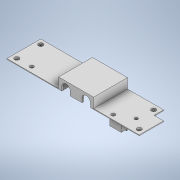
# Autodesk Inventor part: Klapa_kanalpow
Saved by Autodesk Inventor 2022 (Build 260153000, 153)
## iProperties
Created: 2022-09-09
Part Number: Klapa_kanalpow
Material: Ogólny
Document SubType Name: Modeling
Designer: kosak
Density: 1 g/cm^3
Appearance: Domyślna
Author: kosak
Autodesk Inventor part; units mm, degrees
ref_plane "YZ Plane" through (0, 0, 0) normal (1, 0, 0) x (0, 1, 0)
ref_plane "XZ Plane" through (0, 0, 0) normal (0, 1, 0) x (-1, 0, 0)
ref_plane "XY Plane" through (0, 0, 0) normal (0, 0, 1) x (1, 0, 0)
sketch "Szkic1" plane through (0, 0, 0) normal (0, 1, 0) x (-1, 0, 0)
  line L0 (0, 0) -> (174, 0)
  line L1 (174, 0) -> (174, -44.5)
  line L2 (174, -44.5) -> (12.5, -44.5)
  line L3 (0, -32) -> (0, 0)
  line L4 (0, -44.5) -> (12.5, -44.5)
  line L5 (12.5, -44.5) -> (12.5, -32)
  line L6 (12.5, -32) -> (0, -32)
  line L7 (0, -32) -> (0, -44.5)
  dimension "d0" = 174
  dimension "d1" = 44.5
  dimension "d9" = 12.5
  dimension "d10" = 12.5
  constraints: 16 end point, 4 parallel, 2 horizontal, 2 perpendicular
  measures "d0" distance of L1.end L4.start
  measures "d1" distance of L0.end L1.end
  measures "d9" distance of L3.start L5.end
  measures "d10" distance of L2.end L5.end
extrude "Wyciągnięcie proste1" add sketch "Szkic1" along normal blind 1 contours L0 L1 L2 L5 L6 L3
sketch "Szkic2" plane through (0, 0, 0) normal (0, -1, 0) x (1, 0, 0)
  line L0 (-12.5, -44.5) -> (-174, -44.5) projected
  line L1 (0, 0) -> (0, -32) projected
  line L2 (-174, 0) -> (0, 0) projected
  line L3 (-174, -44.5) -> (-174, 0) projected
  line L4 (-171, -41.5) -> (-15, -41.5)
  line L5 (-3, -29.5) -> (-3, -3)
  line L6 (-3, -3) -> (-171, -3)
  line L7 (-171, -3) -> (-171, -41.5)
  line L8 (-12.5, -44.5) -> (-174, -44.5) projected
  line L9 (-15, -41.5) -> (-15, -29.5)
  line L10 (-15, -29.5) -> (-3, -29.5)
  line L11 (-12.5, -32) -> (-12.5, -44.5) projected
  line L12 (0, -32) -> (-12.5, -32) projected
  dimension "d4" = 3
  dimension "d6" = 12
  dimension "d11" = 12
  constraints: 12 end point, 1 other
  measures "d4" distance between parallel lines of L0 L4
  measures "d6" distance of L4.end L9.end
  measures "d11" distance of L9.end L5.start
extrude "Wyciągnięcie proste2" add sketch "Szkic2" along normal blind 2 contours L7 L6 L5 L10 L9 L4
sketch "Szkic4" plane through (0, 1, 0) normal (0, 1, 0) x (1, 0, 0)
  line L0 (-174, 44.5) -> (-174, 0) projected
  line L1 (-174, 22.25) -> (-106, 22.25)
  line L2 (0, 22.25) -> (-60, 22.25)
  line L3 (0, 0) -> (0, 32) projected
  line L4 (-60, 0) -> (-106, 0)
  line L5 (-106, 0) -> (-106, 44.5)
  line L6 (-106, 44.5) -> (-60, 44.5)
  line L7 (-60, 44.5) -> (-60, 0)
  line L8 (-174, 0) -> (0, 0) projected
  line L9 (-12.5, 44.5) -> (-174, 44.5) projected
  dimension "d24" = 60
  dimension "d51" = 68
  constraints: 12 end point, 3 midpoint, 2 collinear, 2 horizontal, 1 parallel, 1 perpendicular, 1 point on line
  measures "d24" distance of L2.start L2.end
  measures "d51" distance of L1.end L1.start
extrude "Wyciągnięcie proste4" add sketch "Szkic4" along normal blind 13 contours L6 L7 L4 L5
sketch "Szkic9" plane through (0, -2, 0) normal (0, -1, 0) x (1, 0, 0)
  line L0 (-60, -44.5) -> (-60, 0) projected
  line L1 (-106, 0) -> (-106, -44.5) projected
  line L2 (-12.5, -44.5) -> (-174, -44.5) projected
  line L3 (-174, 0) -> (0, 0) projected
  line L4 (-104, 0) -> (-104, -44.5)
  line L5 (-62, -44.5) -> (-62, 0)
  line L6 (-12.5, -42.5) -> (-174, -42.5)
  line L7 (-174, -2) -> (0, -2)
  line L8 (-62, -2) -> (-104, -2)
  line L9 (-104, -2) -> (-104, -42.5)
  line L10 (-104, -42.5) -> (-62, -42.5)
  line L11 (-62, -42.5) -> (-62, -2)
  point P0 (-104, -2)
  point P1 (-62, -42.5)
  dimension "d38" = 2
  dimension "d39" = 2
  dimension "d40" = 2
  dimension "d41" = 2
  constraints: 16 end point, 6 parallel, 4 point on line, 1 horizontal, 1 perpendicular
  measures "d38" distance between parallel lines of L1 L4
  measures "d39" distance between parallel lines of L0 L5
  measures "d40" distance between parallel lines of L2 L6
  measures "d41" distance between parallel lines of L3 L7
extrude "Wyciągnięcie proste7" cut sketch "Szkic9" against normal blind 14 contours L6 L4 L7 L5
sketch "Szkic11" plane through (-174, 0, 0) normal (0, 0, 1) x (1, 0, 0)
  line L0 (68, 1) -> (68, 14) projected
  line L1 (114, 1) -> (114, 14) projected
  line L2 (68, 14) -> (114, 14) projected
  line L3 (77.75, 3.9889) -> (77.75, 5.5)
  line L4 (104.25, 5.5) -> (77.75, 5.5)
  circle A0 centre (77.75, 5.5) radius 5.5
  circle A1 centre (104.25, 5.5) radius 5.5
  line L5 (72.25, 5.5) -> (72.25, 0)
  line L6 (161.5, 0) -> (0, 0) projected
  line L7 (83.25, 5.5) -> (83.25, 0)
  line L8 (98.75, 5.5) -> (98.75, 0)
  line L9 (109.75, 5.5) -> (109.75, 0)
  line L10 (0, 0) -> (174, 0) projected
  line L11 (104.25, 5.5) -> (114, 5.5)
  point P0 (77.75, 0)
  dimension "d52" = 9.75
  dimension "d53" = 8.5
  dimension "d54" = 11
  dimension "d55" = 11
  dimension "d59" = 9.75
  constraints: 14 end point, 7 point on line, 4 point on circle, 3 perpendicular, 3 tangent, 2 centre point, 2 coincident, 1 parallel, 1 vertical
  measures "d52" distance between parallel lines of L0 L3
  measures "d53" distance between parallel lines of L2 L4
  measures "d54" diameter of A0
  measures "d55" diameter of A1
  measures "d59" distance of L11.start L11.end
extrude "Wyciągnięcie proste9" cut sketch "Szkic11" against normal blind 2 contours L11 A1 L4 | L4 A1 L11 | A1 L6 L8 | L9 L6 A1 | A0 | L7 L6 A0 | A0 L6 L5
sketch "Szkic12" plane through (0, 1, 0) normal (0, 1, 0) x (1, 0, 0)
  line L0 (-167.5, 44.5) -> (-167.5, 38)
  line L1 (-174, 38) -> (-167.5, 38)
  line L2 (-174, 44.5) -> (-174, 0) projected
  circle A0 centre (-167.5, 38) radius 3
  line L3 (-62, 42.5) -> (-104, 42.5) projected
  line L4 (-171, 3) -> (-171, 41.5) projected
  line L5 (-60, 0) -> (0, 0) projected
  line L6 (-6.5, 0) -> (-6.5, 6.5)
  line L7 (0, 0) -> (0, 32) projected
  line L8 (0, 6.5) -> (-6.5, 6.5)
  circle A1 centre (-6.5, 6.5) radius 3
  line L9 (-12.5, 32) -> (-12.5, 44.5) projected
  line L10 (-12.5, 38) -> (-19, 38)
  line L11 (-12.5, 44.5) -> (-60, 44.5) projected
  line L12 (-19, 44.5) -> (-19, 38)
  circle A2 centre (-19, 38) radius 3
  line L13 (-106, 44.5) -> (-174, 44.5) projected
  line L14 (-174, 6.5) -> (-167.5, 6.5)
  line L15 (-167.5, 0) -> (-167.5, 6.5)
  line L16 (-174, 0) -> (-106, 0) projected
  circle A3 centre (-167.5, 6.5) radius 3
  dimension "d60" = 6.5
  dimension "d61" = 6.5
  dimension "d62" = 6
  dimension "d63" = 6.5
  dimension "d64" = 6.5
  dimension "d65" = 6
  dimension "d66" = 6.5
  dimension "d67" = 6.5
  dimension "d68" = 6
  dimension "d78" = 6.5
  dimension "d79" = 6.5
  dimension "d80" = 6
  constraints: 16 end point, 8 point on line, 4 centre point, 4 coincident, 4 horizontal, 4 vertical
  measures "d60" distance of L1.start L0.end
  measures "d61" distance of L0.end L0.start
  measures "d62" diameter of A0
  measures "d63" distance of L6.end L8.start
  measures "d64" distance of L6.start L6.end
  measures "d65" diameter of A1
  measures "d66" distance of L10.end L10.start
  measures "d67" distance of L12.start L10.end
  measures "d68" diameter of A2
  measures "d78" distance of L14.start L14.end
  measures "d79" distance of L15.start L14.end
  measures "d80" diameter of A3
extrude "Wyciągnięcie proste10" cut sketch "Szkic12" against normal blind 2 contours A0 L1 L0 | L0 L1 A0 | A3 L15 L14 | L14 L15 A3 | A1 L8 L6 | L6 L8 A1 | A2 L12 L10 | L10 L12 A2
sketch "Szkic14" plane through (-167.5, -1, -38) normal (0, 1, 0) x (1, 0, 0)
  circle A0 centre (0, 0) radius 3 projected
  circle A1 centre (0, 0) radius 2
  circle A2 centre (0, -31.5) radius 3 projected
  circle A3 centre (0, -31.5) radius 2
  circle A4 centre (148.5, 0) radius 3 projected
  circle A5 centre (148.5, 0) radius 2
  circle A6 centre (161, -31.5) radius 3 projected
  circle A7 centre (161, -31.5) radius 2
  point P0 (167.5, -38)
  dimension "d81" = 4
  dimension "d82" = 4
  dimension "d83" = 4
  dimension "d84" = 4
  constraints: 4 centre point, 4 coincident
  measures "d81" diameter of A1
  measures "d82" diameter of A3
  measures "d83" diameter of A5
  measures "d84" diameter of A7
extrude "Wyciągnięcie proste12" cut sketch "Szkic14" against normal blind 2 contours A1 | A3 | A5 | A7
sketch "Szkic16" plane through (0, -2, 0) normal (0, -1, 0) x (1, 0, 0)
  line L0 (-3, -3) -> (-62, -3) projected
  line L1 (-62, -41.5) -> (-15, -41.5) projected
  line L2 (-42.6563, -3) -> (-42.6563, -9)
  line L3 (-42.6563, -9) -> (-32.6563, -9)
  line L4 (-32.6563, -9) -> (-47.6563, -9)
  line L5 (-47.6563, -9) -> (-47.6563, -17)
  line L6 (-47.6563, -17) -> (-32.6563, -17)
  line L7 (-32.6563, -17) -> (-32.6563, -9)
  point P0 (0, 0)
  dimension "d93" = 6
  dimension "d94" = 10
  dimension "d95" = 15
  dimension "d96" = 8
  constraints: 12 end point, 2 horizontal, 2 parallel, 1 perpendicular, 1 point on line, 1 vertical
  measures "d93" distance of L2.start L2.end
  measures "d94" distance of L2.end L3.end
  measures "d95" distance of L6.end L5.end
  measures "d96" distance of L5.end L4.end
extrude "Wyciągnięcie proste13" add sketch "Szkic16" along normal blind 15
sketch "Szkic17" plane through (0, -17, 0) normal (0, -1, 0) x (1, 0, 0)
  line L0 (-32.6563, -9) -> (-32.6563, -17) projected
  circle A0 centre (-34.6563, -13.2891) radius 1.5
  line L1 (-34.6563, -13.2891) -> (-45.6563, -13.2891)
  circle A1 centre (-45.6563, -13.2891) radius 1.5
  line L2 (-47.6563, -17) -> (-47.6563, -9) projected
  line L3 (-47.6563, -13.2891) -> (-45.6563, -13.2891)
  point P0 (0, 0)
  dimension "d101" = 3
  dimension "d102" = 11
  dimension "d103" = 3
  dimension "d111" = 2
  constraints: 4 end point, 2 centre point, 2 horizontal, 1 coincident, 1 point on line
  measures "d101" diameter of A0
  measures "d102" distance of L1.end L1.start
  measures "d103" diameter of A1
  measures "d111" distance of L3.start L1.end
extrude "Wyciągnięcie proste14" cut sketch "Szkic17" against normal blind 7
sketch "Szkic18" plane through (0, -17, 0) normal (0, -1, 0) x (1, 0, 0)
  line L0 (-47.6563, -17) -> (-47.6563, -9) projected
  line L1 (-32.6563, -17) -> (-32.6563, -9) projected
  line L2 (-32.6563, -17) -> (-32.6563, -16.2)
  line L3 (-47.6563, -16.2) -> (-47.6563, -17)
  line L4 (-47.6563, -17) -> (-32.6563, -17) projected
  line L5 (-47.6563, -16.2) -> (-43.6563, -16.2)
  line L6 (-43.6563, -16.2) -> (-43.6563, -17)
  line L7 (-43.6563, -17) -> (-47.6563, -17)
  line L8 (-47.6563, -17) -> (-47.6563, -16.2)
  line L9 (-32.6563, -17) -> (-36.6563, -17)
  line L10 (-36.6563, -17) -> (-36.6563, -16.2)
  line L11 (-36.6563, -16.2) -> (-32.6563, -16.2)
  line L12 (-32.6563, -16.2) -> (-32.6563, -17)
  point P0 (0, 0)
  point P1 (-36.6563, -17)
  dimension "d109" = 4
  dimension "d110" = 4
  constraints: 20 end point, 5 parallel, 3 point on line, 2 horizontal, 2 perpendicular
  measures "d109" distance of L6.end L7.end
  measures "d110" distance of L10.end L11.end
extrude "Wyciągnięcie proste15" add sketch "Szkic18" along normal blind 2
sketch "Szkic19" plane through (0, 1, 0) normal (0, 1, 0) x (1, 0, 0)
  line L0 (0, 0) -> (0, 32) projected
  line L1 (0, 16.5) -> (-20.402, 16.5)
  line L2 (-60, 0) -> (0, 0) projected
  line L3 (-20.402, 0) -> (-20.402, 16.5)
  circle A0 centre (-20.402, 16.5) radius 2.1
  dimension "d112" = 20.402
  dimension "d113" = 16.5
  dimension "d114" = 4.2
  constraints: 4 end point, 2 point on line, 1 centre point, 1 coincident, 1 perpendicular, 1 vertical
  measures "d112" distance of L1.end L1.start
  measures "d113" distance of L3.start L1.end
  measures "d114" diameter of A0
extrude "Wyciągnięcie proste16" cut sketch "Szkic19" against normal blind 4 contours A0 L3 L1 | L1 L3 A0
sketch "Szkic20" plane through (0, 1, 0) normal (0, 1, 0) x (1, 0, 0)
  line L0 (-174, 44.5) -> (-174, 0) projected
  line L1 (-174, 7) -> (-148.327, 7)
  line L2 (-171, 3) -> (-104, 3) projected
  line L3 (-174, 0) -> (-101.75, 0) projected
  line L4 (-148.327, 0) -> (-148.327, 7)
  circle A0 centre (-148.327, 7) radius 2.5
  point P0 (0, 0)
  dimension "d117" = 25.673
  dimension "d118" = 7
  dimension "d119" = 5
  constraints: 4 end point, 2 point on line, 1 centre point, 1 coincident, 1 parallel, 1 perpendicular
  measures "d117" distance of L1.start L1.end
  measures "d118" distance of L1.end L4.start
  measures "d119" diameter of A0
extrude "Wyciągnięcie proste17" cut sketch "Szkic20" against normal blind 4 contours A0 L4 L1 | L1 L4 A0
sketch "Szkic21" plane through (0, -2, 0) normal (0, -1, 0) x (1, 0, 0)
  line L0 (-47.6563, -9) -> (-32.6563, -9) projected
  line L1 (-40.1563, -9) -> (-40.1563, -7)
  line L2 (-40.1563, -7) -> (-40.8563, -7)
  line L3 (-40.1563, -7) -> (-39.4563, -7)
  line L4 (-39.4563, -7) -> (-39.3563, -7)
  line L5 (-40.1563, -7) -> (-40.1563, -5)
  circle A0 centre (-40.1563, -6) radius 2.5
  point P0 (0, 0)
  dimension "d122" = 2
  dimension "d123" = 0.7
  dimension "d124" = 0.7
  dimension "d209" = 2
  dimension "d210" = 5
  constraints: 10 end point, 3 horizontal, 2 midpoint, 2 vertical, 1 centre point
  measures "d122" distance of L1.start L1.end
  measures "d123" distance of L2.end L1.end
  measures "d124" distance of L1.end L3.end
  measures "d209" distance of L1.end L5.end
  measures "d210" diameter of A0
thread "Gwint1" size "M4x0.7" class "6H" standard "ANSI Metric M Profile" full length
thread "Gwint2" size "M4x0.7" class "6H" standard "ANSI Metric M Profile" full length
thread "Gwint3" size "M4x0.7" class "6H" standard "ANSI Metric M Profile" full length
thread "Gwint4" size "M4x0.7" class "6H" standard "ANSI Metric M Profile" full length
sketch "Szkic23" plane through (-167.5, -2, -38) normal (-1, 0, 0) x (0, 0, 1)
  line L0 (2, 0) -> (2, 1)
  line L1 (2, 1) -> (1.481, 1)
  line L2 (1.481, 1) -> (1.481, 0)
  line L3 (1.481, 0) -> (2, 0)
  line L4 (0, -23.6) -> (0, 22.6) projected
  constraints: 8 end point
revolve "Obrót1" add sketch "Szkic23" angle 360 about axis through (-167.5, -2, -38) along (0, 1, 0) separate body
sketch "Szkic22" plane through (-167.5, -2, -36) normal (1, 0, 0) x (0, 1, 0)
  line L0 (-0.4084, -0.0356) -> (-0.3501, -0.0356) construction
  line L1 (0.0582, -0.4838) -> (-0.0001, -0.5959) construction
  line L2 (-0.7001, -0.5959) -> (-0.7584, -0.4838) construction
  line L3 (-0.2918, -0.0356) -> (-0.3501, 0.0765) construction
  line L4 (-0.3501, 0.0765) -> (-0.4084, -0.0356) construction
  line L5 (-0.7001, -0.5959) -> (-0.6418, -0.4838) construction
  line L6 (-0.2918, -0.0356) -> (-0.0584, -0.4838)
  line L7 (-0.7584, -0.4838) -> (-0.6418, -0.4838) construction
  arc A0 (-0.7584, -0.4838) -> (-0.7001, -0.5192) centre (-0.7001, -0.4534) ccw construction
  line L8 (0.0582, -0.4838) -> (-0.0584, -0.4838) construction
  line L9 (-0.7001, -0.5959) -> (-0.7001, -0.4838) construction
  line L10 (-0.0001, -0.5959) -> (-0.0001, -0.4838) construction
  line L11 (-0.3501, 0.0765) -> (-0.3501, -0.0002) construction
  line L12 (-0.7001, -0.5192) -> (-0.0001, -0.5192)
  arc A1 (-0.7001, -0.5192) -> (-0.6418, -0.4838) centre (-0.7001, -0.4534) ccw
  line L13 (-0.0584, -0.4838) -> (-0.0001, -0.5959) construction
  line L14 (-0.6418, -0.4838) -> (-0.4084, -0.0356)
  line L15 (-0.0001, -0.0002) -> (-0.0001, 0.0177)
  line L16 (-0.0001, 0.0177) -> (-0.0001, -0.0002)
  line L17 (-0.0001, -0.0002) -> (0.0334, -0.0002)
  arc A2 (-0.0584, -0.4838) -> (-0.0001, -0.5192) centre (-0.0001, -0.4534) ccw
  arc A3 (-0.0001, -0.5192) -> (0.0582, -0.4838) centre (-0.0001, -0.4534) ccw construction
  arc A4 (-0.3501, -0.0002) -> (-0.4084, -0.0356) centre (-0.3501, -0.0659) ccw
  arc A5 (-0.2918, -0.0356) -> (-0.3501, -0.0002) centre (-0.3501, -0.0659) ccw
  line L18 (-0.3501, -0.0002) -> (-0.3501, -0.0356) construction
  line L19 (-0.3501, -0.0356) -> (-0.2918, -0.0356) construction
  dimension "d137" = 55
  dimension "d138" = 0.1121
  dimension "d139" = 0.1121
  dimension "Szkic22_ThreadOffset" = 0
  dimension "Szkic22_MajorRadius" = 0.519
  dimension "d142" = 0.7
  dimension "Szkic22_MinorRadius" = 0
  constraints: 40 end point, 12 point on circle, 10 parallel, 8 tangent, 6 centre point, 6 collinear, 2 midpoint, 2 point on line, 1 horizontal, 1 perpendicular, 3 other
  measures "d137" angle of L6 L14
  measures "d138" distance of L3.end L0.end
  measures "d139" distance of L1.end L10.end
  measures "Szkic22_ThreadOffset" distance between parallel lines of L15 L10
  measures "Szkic22_MajorRadius" distance from line of L12 L15.start
  measures "d142" distance from line of L1.end L9
  measures "Szkic22_MinorRadius" distance edge to line of A5 L17
coil "Zwój1" sketch "Szkic22" operation cut axis through (-167.5, -2, -38) along (0, 1, 0) pitch 0.7007 turns 3.425146 hand right bodies 2
sketch "Szkic25" plane through (-167.5, -2, -6.5) normal (-1, 0, 0) x (0, 0, 1)
  line L0 (2, 0) -> (2, 1)
  line L1 (2, 1) -> (1.481, 1)
  line L2 (1.481, 1) -> (1.481, 0)
  line L3 (1.481, 0) -> (2, 0)
  line L4 (0, -23.6) -> (0, 22.6) projected
  constraints: 8 end point
revolve "Obrót2" add sketch "Szkic25" angle 360 about axis through (-167.5, -2, -6.5) along (0, 1, 0) separate body
sketch "Szkic24" plane through (-167.5, -2, -4.5) normal (1, 0, 0) x (0, 1, 0)
  line L0 (-0.4084, -0.0356) -> (-0.3501, -0.0356) construction
  line L1 (0.0582, -0.4838) -> (-0.0001, -0.5959) construction
  line L2 (-0.7001, -0.5959) -> (-0.7584, -0.4838) construction
  line L3 (-0.2918, -0.0356) -> (-0.3501, 0.0765) construction
  line L4 (-0.3501, 0.0765) -> (-0.4084, -0.0356) construction
  line L5 (-0.7001, -0.5959) -> (-0.6418, -0.4838) construction
  line L6 (-0.2918, -0.0356) -> (-0.0584, -0.4838)
  line L7 (-0.7584, -0.4838) -> (-0.6418, -0.4838) construction
  arc A0 (-0.7584, -0.4838) -> (-0.7001, -0.5192) centre (-0.7001, -0.4534) ccw construction
  line L8 (0.0582, -0.4838) -> (-0.0584, -0.4838) construction
  line L9 (-0.7001, -0.5959) -> (-0.7001, -0.4838) construction
  line L10 (-0.0001, -0.5959) -> (-0.0001, -0.4838) construction
  line L11 (-0.3501, 0.0765) -> (-0.3501, -0.0002) construction
  line L12 (-0.7001, -0.5192) -> (-0.0001, -0.5192)
  arc A1 (-0.7001, -0.5192) -> (-0.6418, -0.4838) centre (-0.7001, -0.4534) ccw
  line L13 (-0.0584, -0.4838) -> (-0.0001, -0.5959) construction
  line L14 (-0.6418, -0.4838) -> (-0.4084, -0.0356)
  line L15 (-0.0001, -0.0002) -> (-0.0001, 0.0177)
  line L16 (-0.0001, 0.0177) -> (-0.0001, -0.0002)
  line L17 (-0.0001, -0.0002) -> (0.0334, -0.0002)
  arc A2 (-0.0584, -0.4838) -> (-0.0001, -0.5192) centre (-0.0001, -0.4534) ccw
  arc A3 (-0.0001, -0.5192) -> (0.0582, -0.4838) centre (-0.0001, -0.4534) ccw construction
  arc A4 (-0.3501, -0.0002) -> (-0.4084, -0.0356) centre (-0.3501, -0.0659) ccw
  arc A5 (-0.2918, -0.0356) -> (-0.3501, -0.0002) centre (-0.3501, -0.0659) ccw
  line L18 (-0.3501, -0.0002) -> (-0.3501, -0.0356) construction
  line L19 (-0.3501, -0.0356) -> (-0.2918, -0.0356) construction
  dimension "d155" = 55
  dimension "d156" = 0.1121
  dimension "d157" = 0.1121
  dimension "Szkic24_ThreadOffset" = 0
  dimension "Szkic24_MajorRadius" = 0.519
  dimension "d160" = 0.7
  dimension "Szkic24_MinorRadius" = 0
  constraints: 40 end point, 12 point on circle, 10 parallel, 8 tangent, 6 centre point, 6 collinear, 2 midpoint, 2 point on line, 1 horizontal, 1 perpendicular, 3 other
  measures "d155" angle of L6 L14
  measures "d156" distance of L3.end L0.end
  measures "d157" distance of L1.end L10.end
  measures "Szkic24_ThreadOffset" distance between parallel lines of L15 L10
  measures "Szkic24_MajorRadius" distance from line of L12 L15.start
  measures "d160" distance from line of L1.end L9
  measures "Szkic24_MinorRadius" distance edge to line of A5 L17
coil "Zwój2" sketch "Szkic24" operation cut axis through (-167.5, -2, -6.5) along (0, 1, 0) pitch 0.7007 turns 3.425146 hand right bodies 3
sketch "Szkic27" plane through (-19, -2, -38) normal (-1, 0, 0) x (0, 0, 1)
  line L0 (2, 0) -> (2, 1)
  line L1 (2, 1) -> (1.481, 1)
  line L2 (1.481, 1) -> (1.481, 0)
  line L3 (1.481, 0) -> (2, 0)
  line L4 (0, -23.6) -> (0, 22.6) projected
  constraints: 8 end point
revolve "Obrót3" add sketch "Szkic27" angle 360 about axis through (-19, -2, -38) along (0, 1, 0) separate body
sketch "Szkic26" plane through (-19, -2, -36) normal (1, 0, 0) x (0, 1, 0)
  line L0 (-0.4084, -0.0356) -> (-0.3501, -0.0356) construction
  line L1 (0.0582, -0.4838) -> (-0.0001, -0.5959) construction
  line L2 (-0.7001, -0.5959) -> (-0.7584, -0.4838) construction
  line L3 (-0.2918, -0.0356) -> (-0.3501, 0.0765) construction
  line L4 (-0.3501, 0.0765) -> (-0.4084, -0.0356) construction
  line L5 (-0.7001, -0.5959) -> (-0.6418, -0.4838) construction
  line L6 (-0.2918, -0.0356) -> (-0.0584, -0.4838)
  line L7 (-0.7584, -0.4838) -> (-0.6418, -0.4838) construction
  arc A0 (-0.7584, -0.4838) -> (-0.7001, -0.5192) centre (-0.7001, -0.4534) ccw construction
  line L8 (0.0582, -0.4838) -> (-0.0584, -0.4838) construction
  line L9 (-0.7001, -0.5959) -> (-0.7001, -0.4838) construction
  line L10 (-0.0001, -0.5959) -> (-0.0001, -0.4838) construction
  line L11 (-0.3501, 0.0765) -> (-0.3501, -0.0002) construction
  line L12 (-0.7001, -0.5192) -> (-0.0001, -0.5192)
  arc A1 (-0.7001, -0.5192) -> (-0.6418, -0.4838) centre (-0.7001, -0.4534) ccw
  line L13 (-0.0584, -0.4838) -> (-0.0001, -0.5959) construction
  line L14 (-0.6418, -0.4838) -> (-0.4084, -0.0356)
  line L15 (-0.0001, -0.0002) -> (-0.0001, 0.0177)
  line L16 (-0.0001, 0.0177) -> (-0.0001, -0.0002)
  line L17 (-0.0001, -0.0002) -> (0.0334, -0.0002)
  arc A2 (-0.0584, -0.4838) -> (-0.0001, -0.5192) centre (-0.0001, -0.4534) ccw
  arc A3 (-0.0001, -0.5192) -> (0.0582, -0.4838) centre (-0.0001, -0.4534) ccw construction
  arc A4 (-0.3501, -0.0002) -> (-0.4084, -0.0356) centre (-0.3501, -0.0659) ccw
  arc A5 (-0.2918, -0.0356) -> (-0.3501, -0.0002) centre (-0.3501, -0.0659) ccw
  line L18 (-0.3501, -0.0002) -> (-0.3501, -0.0356) construction
  line L19 (-0.3501, -0.0356) -> (-0.2918, -0.0356) construction
  dimension "d173" = 55
  dimension "d174" = 0.1121
  dimension "d175" = 0.1121
  dimension "Szkic26_ThreadOffset" = 0
  dimension "Szkic26_MajorRadius" = 0.519
  dimension "d178" = 0.7
  dimension "Szkic26_MinorRadius" = 0
  constraints: 40 end point, 12 point on circle, 10 parallel, 8 tangent, 6 centre point, 6 collinear, 2 midpoint, 2 point on line, 1 horizontal, 1 perpendicular, 3 other
  measures "d173" angle of L6 L14
  measures "d174" distance of L3.end L0.end
  measures "d175" distance of L1.end L10.end
  measures "Szkic26_ThreadOffset" distance between parallel lines of L15 L10
  measures "Szkic26_MajorRadius" distance from line of L12 L15.start
  measures "d178" distance from line of L1.end L9
  measures "Szkic26_MinorRadius" distance edge to line of A5 L17
coil "Zwój3" sketch "Szkic26" operation cut axis through (-19, -2, -38) along (0, 1, 0) pitch 0.7007 turns 3.425146 hand right bodies 4
sketch "Szkic29" plane through (-6.5, -2, -6.5) normal (-1, 0, 0) x (0, 0, 1)
  line L0 (2, 0) -> (2, 1)
  line L1 (2, 1) -> (1.481, 1)
  line L2 (1.481, 1) -> (1.481, 0)
  line L3 (1.481, 0) -> (2, 0)
  line L4 (0, -23.6) -> (0, 22.6) projected
  constraints: 8 end point
revolve "Obrót4" add sketch "Szkic29" angle 360 about axis through (-6.5, -2, -6.5) along (0, 1, 0) separate body
sketch "Szkic28" plane through (-6.5, -2, -4.5) normal (1, 0, 0) x (0, 1, 0)
  line L0 (-0.4084, -0.0356) -> (-0.3501, -0.0356) construction
  line L1 (0.0582, -0.4838) -> (-0.0001, -0.5959) construction
  line L2 (-0.7001, -0.5959) -> (-0.7584, -0.4838) construction
  line L3 (-0.2918, -0.0356) -> (-0.3501, 0.0765) construction
  line L4 (-0.3501, 0.0765) -> (-0.4084, -0.0356) construction
  line L5 (-0.7001, -0.5959) -> (-0.6418, -0.4838) construction
  line L6 (-0.2918, -0.0356) -> (-0.0584, -0.4838)
  line L7 (-0.7584, -0.4838) -> (-0.6418, -0.4838) construction
  arc A0 (-0.7584, -0.4838) -> (-0.7001, -0.5192) centre (-0.7001, -0.4534) ccw construction
  line L8 (0.0582, -0.4838) -> (-0.0584, -0.4838) construction
  line L9 (-0.7001, -0.5959) -> (-0.7001, -0.4838) construction
  line L10 (-0.0001, -0.5959) -> (-0.0001, -0.4838) construction
  line L11 (-0.3501, 0.0765) -> (-0.3501, -0.0002) construction
  line L12 (-0.7001, -0.5192) -> (-0.0001, -0.5192)
  arc A1 (-0.7001, -0.5192) -> (-0.6418, -0.4838) centre (-0.7001, -0.4534) ccw
  line L13 (-0.0584, -0.4838) -> (-0.0001, -0.5959) construction
  line L14 (-0.6418, -0.4838) -> (-0.4084, -0.0356)
  line L15 (-0.0001, -0.0002) -> (-0.0001, 0.0177)
  line L16 (-0.0001, 0.0177) -> (-0.0001, -0.0002)
  line L17 (-0.0001, -0.0002) -> (0.0334, -0.0002)
  arc A2 (-0.0584, -0.4838) -> (-0.0001, -0.5192) centre (-0.0001, -0.4534) ccw
  arc A3 (-0.0001, -0.5192) -> (0.0582, -0.4838) centre (-0.0001, -0.4534) ccw construction
  arc A4 (-0.3501, -0.0002) -> (-0.4084, -0.0356) centre (-0.3501, -0.0659) ccw
  arc A5 (-0.2918, -0.0356) -> (-0.3501, -0.0002) centre (-0.3501, -0.0659) ccw
  line L18 (-0.3501, -0.0002) -> (-0.3501, -0.0356) construction
  line L19 (-0.3501, -0.0356) -> (-0.2918, -0.0356) construction
  dimension "d191" = 55
  dimension "d192" = 0.1121
  dimension "d193" = 0.1121
  dimension "Szkic28_ThreadOffset" = 0
  dimension "Szkic28_MajorRadius" = 0.519
  dimension "d196" = 0.7
  dimension "Szkic28_MinorRadius" = 0
  constraints: 40 end point, 12 point on circle, 10 parallel, 8 tangent, 6 centre point, 6 collinear, 2 midpoint, 2 point on line, 1 horizontal, 1 perpendicular, 3 other
  measures "d191" angle of L6 L14
  measures "d192" distance of L3.end L0.end
  measures "d193" distance of L1.end L10.end
  measures "Szkic28_ThreadOffset" distance between parallel lines of L15 L10
  measures "Szkic28_MajorRadius" distance from line of L12 L15.start
  measures "d196" distance from line of L1.end L9
  measures "Szkic28_MinorRadius" distance edge to line of A5 L17
coil "Zwój4" sketch "Szkic28" operation cut axis through (-6.5, -2, -6.5) along (0, 1, 0) pitch 0.7007 turns 3.425146 hand right bodies 5
extrude "Wyciągnięcie proste19" cut sketch "Szkic21" against normal blind 10 bodies 1
equation "\"d63\" = d61"
equation "\"d64\" = d60"
equation "\"d65\" = d62"
equation "\"d66\" = d64"
equation "\"d67\" = d61"
equation "\"d68\" = d65"
equation "\"d82\" = d81"
equation "\"d83\" = d81"
equation "\"d84\" = d83"
equation "\"d137\" = d144"
equation "\"d138\" = 0.160083 * Szkic22_Pitch"
equation "\"d139\" = 0.160083 * Szkic22_Pitch"
equation "\"d142\" = Szkic22_Pitch"
equation "\"d155\" = d162"
equation "\"d156\" = 0.160083 * Szkic24_Pitch"
equation "\"d157\" = 0.160083 * Szkic24_Pitch"
equation "\"d160\" = Szkic24_Pitch"
equation "\"d173\" = d180"
equation "\"d174\" = 0.160083 * Szkic26_Pitch"
equation "\"d175\" = 0.160083 * Szkic26_Pitch"
equation "\"d178\" = Szkic26_Pitch"
equation "\"d191\" = d198"
equation "\"d192\" = 0.160083 * Szkic28_Pitch"
equation "\"d193\" = 0.160083 * Szkic28_Pitch"
equation "\"d196\" = Szkic28_Pitch"
equation "\"d144\" = 55deg"
equation "\"Szkic22_Pitch\" = 0.7"
equation "\"d162\" = 55deg"
equation "\"Szkic24_Pitch\" = 0.7"
equation "\"d180\" = 55deg"
equation "\"Szkic26_Pitch\" = 0.7"
equation "\"d198\" = 55deg"
equation "\"Szkic28_Pitch\" = 0.7"
